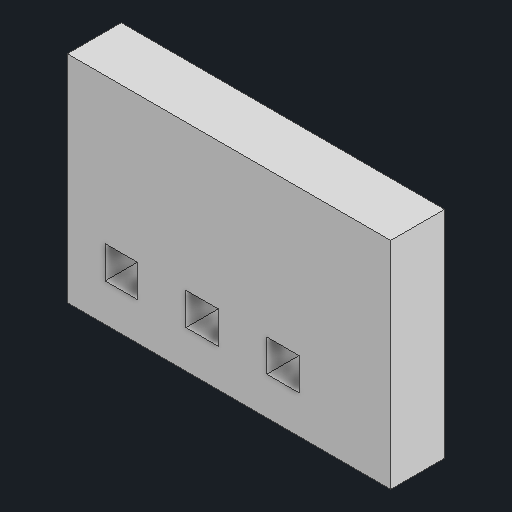
# Autodesk Inventor part: 21_pocket_rect
Saved by Autodesk Inventor 2027 (Build 310192060, 192F)
## iProperties
Created: 2026-07-12
Part Number: 21_pocket_rect
Material: Generic
Document SubType Name: Modeling
Designer: vmiguel
Density: 1 g/cm^3
Appearance: Default
Author: vmiguel
Autodesk Inventor part; units mm, degrees
ref_plane "YZ Plane" through (0, 0, 0) normal (1, 0, 0) x (0, 1, 0)
ref_plane "XZ Plane" through (0, 0, 0) normal (0, 1, 0) x (-1, 0, 0)
ref_plane "XY Plane" through (0, 0, 0) normal (0, 0, 1) x (1, 0, 0)
sketch "Sketch1" plane through (0, 0, 0) normal (0, 0, 1) x (1, 0, 0)
  line L0 (0, 0) -> (60, 0)
  line L1 (60, 0) -> (60, 40)
  line L2 (60, 40) -> (0, 40)
  line L3 (0, 40) -> (0, 0)
  constraints: 8 end point, 2 parallel, 1 horizontal, 1 perpendicular
extrude "Extrusion1" add sketch "Sketch1" along normal blind 10
sketch "Sketch2" plane through (0, 0, 0) normal (0, 0, 1) x (1, 0, 0)
  line L0 (7, 7) -> (13, 7)
  line L1 (13, 7) -> (13, 13)
  line L2 (13, 13) -> (7, 13)
  line L3 (7, 13) -> (7, 7)
  constraints: 8 end point, 2 parallel, 1 horizontal, 1 perpendicular
extrude "Extrusion2" cut sketch "Sketch2" along normal blind 10
pattern_linear "Rectangular Pattern1" count 3 spacing 15 along (1, 0, 0) of "Extrusion2"
body "Solid1"
